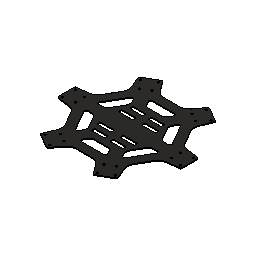
F550 Top Plate v11 (Autodesk Fusion 360 design; units mm, degrees)
Autodesk Fusion 360 part; units mm, degrees
sketch "Sketch1" plane through (0, 0, 0) normal (0, 0, 1) x (1, 0, 0)
  circle A0 centre (0, 0) radius 275 construction
  line L0 (-110, -15.85) -> (-110, 15.85)
  circle A1 centre (-105, 11.7505) radius 1.75
  circle A2 centre (-105, -11.7505) radius 1.75
  line L1 (-105, 11.7505) -> (-105, -11.7505) construction
  line L2 (0, 0) -> (-67.55, 39)
  line L3 (0, 0) -> (-67.55, -39)
  line L4 (0, 0) -> (-105, 0) construction
  line L5 (-110, -15.85) -> (-87.3993, -18.5941)
  line L6 (-67.55, -39) -> (-74.3532, -27.2165)
  arc A3 (-74.3532, -27.2165) -> (-87.3993, -18.5941) centre (-89.5086, -35.9665) ccw
  line L7 (-110, 15.85) -> (-87.3993, 18.5941)
  arc A4 (-87.3993, 18.5941) -> (-74.3532, 27.2165) centre (-89.5086, 35.9665) ccw
  line L8 (-67.55, 39) -> (-74.3532, 27.2165)
  circle A5 centre (-85.5, 8) radius 1.75
  circle A6 centre (-85.5, -8) radius 1.75
  line L9 (-85.5, -8) -> (-85.5, 8)
  line L10 (-54.5596, 31.5) -> (-64.5596, 14.1795)
  line L11 (-41.5692, 24) -> (-46.9504, 14.6795)
  line L12 (-61.9615, 9.6795) -> (-55.6107, 9.6795)
  arc A7 (-55.6107, 9.6795) -> (-46.9504, 14.6795) centre (-55.6107, 19.6795) ccw
  arc A8 (-64.5596, 14.1795) -> (-61.9615, 9.6795) centre (-61.9615, 12.6795) ccw
  line L13 (-54.5596, -31.5) -> (-64.5596, -14.1795)
  arc A9 (-61.9615, -9.6795) -> (-64.5596, -14.1795) centre (-61.9615, -12.6795) ccw
  line L14 (-61.9615, -9.6795) -> (-55.6107, -9.6795)
  arc A10 (-46.9504, -14.6795) -> (-55.6107, -9.6795) centre (-55.6107, -19.6795) ccw
  line L15 (-41.5692, -24) -> (-46.9504, -14.6795)
  point P0 (-110, 0)
  point P1 (-105, 0)
  point P2 (-275, 0)
  point P3 (-85.5, 0)
  point P4 (-107, -10)
  point P5 (-107, 10)
  point P6 (-107, 0)
  dimension "d1" = 550
  dimension "d2" = 23.501
  dimension "d3" = 5
  dimension "d5" = 170
  dimension "d6" = 3.5
  dimension "d7" = 31.7
  dimension "d8" = 30
  dimension "d9" = 30
  dimension "d10" = 78
  dimension "d11" = 16
  dimension "d12" = 19.5
  dimension "d13" = 20
  dimension "d23" = 3
  dimension "d24" = 10
  dimension "d25" = 15
  dimension "d26" = 60
  dimension "d28" = 15
  dimension "d29" = 20
  dimension "d30" = 105
  dimension "d31" = 23.359
  dimension "d44" = 17.5
  constraint coincident A0.centre L2.start
  constraint vertical L0
  constraint midpoint L0 P0
  constraint horizontal A0.centre P0
  constraint vertical A1.centre A2.centre
  constraint coincident A1.centre L1.start
  constraint coincident A2.centre L1.end
  constraint midpoint L1 P1
  constraint coincident A0 P2
  constraint horizontal A0.centre P2
  constraint equal A1 A2
  constraint coincident P1 L4.end
  constraint horizontal A0.centre P1
  constraint equal L2 L3
  constraint perpendicular L3 L6
  constraint tangent L6 A3
  constraint tangent L5 A3
  constraint symmetric L0.start L4 L0.end
  constraint symmetric L3.end L4 L2.end
  constraint symmetric L4 L5.end L7.end
  constraint symmetric L4 L6.end A4.end
  constraint symmetric L4 A3 A4
  constraint equal A5 A6
  constraint equal A1 A5
  constraint coincident A6.centre L9.start
  constraint coincident A5.centre L9.end
  constraint vertical L9
  constraint midpoint L9 P3
  constraint coincident L4 P3
  constraint coincident L2 L10.start
  constraint perpendicular L2 L10
  constraint coincident L2 L11.start
  constraint perpendicular L2 L11
  constraint tangent L11 A7
  constraint tangent L12 A8
  constraint tangent L10 A8
  constraint tangent L12 A7
  constraint symmetric L4 L10.start L13.start
  constraint symmetric L4 L10.end L13.end
  constraint symmetric L4 L11.start L15.start
  constraint symmetric L4 L11.end A10.start
  constraint symmetric L4 L12.start A9.start
  constraint symmetric L4 L12.end L14.end
  constraint symmetric L4 A7 A10
  constraint symmetric L4 A8 A9
  constraint coincident L4 P6
  measures "d1" diameter of A0
  measures "d2" distance of A1.centre A2.centre
  measures "d3" distance of L0 L1
  measures "d5" distance of L1 P2
  measures "d6" diameter of A1
  measures "d7" distance of L0.start L0.end
  measures "d8" angle of L3 L4
  measures "d9" angle of L2 L4
  measures "d10" distance of A0.centre L2.end
  measures "d11" distance of A6.centre A5.centre
  measures "d12" distance of L1 L9
  measures "d13" distance of P4 P5
  measures "d23" radius of A8
  measures "d24" radius of A7
  measures "d25" distance of L10 L11
  measures "d26" angle of L10 L12
  measures "d28" distance of L8 L10
  measures "d29" distance of L2 L10.end
  measures "d30" distance of L1 A0.centre
  measures "d44" radius of A4
extrude "Extrude1" add sketch "Sketch1" along normal blind 1.5 contours L0 L2 L3 L5 L6 A3 L7 A4 L8 L10 L11 L12 A7 A8 L13 A9 L14 A10 L15 makes body 1
fillet "Fillet1" radius 2 2 edges at (-110, 15.85, 0.75) (-110, -15.85, 0.75) on bodies 1
pattern_circular "C-Pattern1" count 6 over 360 about axis through (0, 0, 1.75) along (0, 0, 1) of bodies 1 makes body 2 at (-15.6501, -27.1068, 0) makes body 3 at (15.6501, -27.1068, 0) makes body 4 at (31.3003, 0, 1.5) makes body 5 at (15.6501, 27.1068, 0) makes body 6 at (-15.6501, 27.1068, 0)
combine "Combine1" operation add target body 1 tool bodies 2 3 4 5 6
sketch "Sketch2" plane through (0, 0, 1.5) normal (0, 0, 1) x (-1, 0, 0)
  line L0 (36.188, -33.3205) -> (46.9504, -14.6795)
  arc A0 (55.6107, -9.6795) -> (46.9504, -14.6795) centre (55.6107, -19.6795) ccw
  line L1 (55.6107, -9.6795) -> (61.9615, -9.6795)
  arc A1 (64.5596, -14.1795) -> (61.9615, -9.6795) centre (61.9615, -12.6795) ccw
  line L2 (64.5596, -14.1795) -> (44.5596, -48.8205)
  arc A2 (39.3634, -48.8205) -> (44.5596, -48.8205) centre (41.9615, -47.3205) ccw
  line L3 (39.3634, -48.8205) -> (36.188, -43.3205)
  arc A3 (36.188, -33.3205) -> (36.188, -43.3205) centre (44.8483, -38.3205) ccw
  line L4 (-10.7624, -48) -> (10.7624, -48)
  arc A4 (19.4226, -53) -> (10.7624, -48) centre (10.7624, -58) ccw
  line L5 (19.4226, -53) -> (22.5981, -58.5)
  arc A5 (20, -63) -> (22.5981, -58.5) centre (20, -60) ccw
  line L6 (20, -63) -> (-20, -63)
  circle A6 centre (49.6782, -70.0452) radius 1.75
  circle A7 centre (35.8218, -78.0452) radius 1.75
  circle A8 centre (62.6762, -85.0574) radius 1.75
  circle A9 centre (42.3238, -96.8079) radius 1.75
  line L7 (-13.6064, -78) -> (13.6064, -78)
  arc A10 (27.5967, -84.9871) -> (13.6064, -78) centre (13.6064, -95.5) ccw
  line L8 (27.5967, -84.9871) -> (40.2091, -101.7713)
  arc A11 (40.2091, -101.7713) -> (42.808, -102.3019) centre (41.808, -100.5698) ccw
  line L9 (42.808, -102.3019) -> (67.192, -88.2237)
  arc A12 (67.192, -88.2237) -> (68.032, -85.7077) centre (66.192, -86.4917) ccw
  line L10 (68.032, -85.7077) -> (59.8026, -66.393)
  arc A13 (60.7468, -50.7835) -> (59.8026, -66.393) centre (75.9022, -59.5335) ccw
  line L11 (60.7468, -50.7835) -> (74.3532, -27.2165)
  arc A14 (87.3993, -18.5941) -> (74.3532, -27.2165) centre (89.5086, -35.9665) ccw
  line L12 (87.3993, -18.5941) -> (108.2411, -16.0636)
  arc A15 (108.2411, -16.0636) -> (110, -14.0781) centre (108, -14.0781) ccw
  line L13 (110, -14.0781) -> (110, 14.0781)
  arc A16 (110, 14.0781) -> (108.2411, 16.0636) centre (108, 14.0781) ccw
  line L14 (108.2411, 16.0636) -> (87.3993, 18.5941)
  arc A17 (74.3532, 27.2165) -> (87.3993, 18.5941) centre (89.5086, 35.9665) ccw
  line L15 (74.3532, 27.2165) -> (60.7468, 50.7835)
  arc A18 (59.8026, 66.393) -> (60.7468, 50.7835) centre (75.9022, 59.5335) ccw
  line L16 (59.8026, 66.393) -> (68.032, 85.7077)
  arc A19 (68.032, 85.7077) -> (67.192, 88.2237) centre (66.192, 86.4917) ccw
  line L17 (67.192, 88.2237) -> (42.808, 102.3019)
  arc A20 (42.808, 102.3019) -> (40.2091, 101.7713) centre (41.808, 100.5698) ccw
  line L18 (40.2091, 101.7713) -> (27.5967, 84.9871)
  arc A21 (13.6064, 78) -> (27.5967, 84.9871) centre (13.6064, 95.5) ccw
  line L19 (13.6064, 78) -> (-13.6064, 78)
  arc A22 (-27.5967, 84.9871) -> (-13.6064, 78) centre (-13.6064, 95.5) ccw
  line L20 (-27.5967, 84.9871) -> (-40.2091, 101.7713)
  arc A23 (-40.2091, 101.7713) -> (-42.808, 102.3019) centre (-41.808, 100.5698) ccw
  line L21 (-42.808, 102.3019) -> (-67.192, 88.2237)
  arc A24 (-67.192, 88.2237) -> (-68.032, 85.7077) centre (-66.192, 86.4917) ccw
  line L22 (-68.032, 85.7077) -> (-59.8026, 66.393)
  arc A25 (-60.7468, 50.7835) -> (-59.8026, 66.393) centre (-75.9022, 59.5335) ccw
  line L23 (-60.7468, 50.7835) -> (-74.3532, 27.2165)
  arc A26 (-87.3993, 18.5941) -> (-74.3532, 27.2165) centre (-89.5086, 35.9665) ccw
  line L24 (-87.3993, 18.5941) -> (-108.2411, 16.0636)
  arc A27 (-108.2411, 16.0636) -> (-110, 14.0781) centre (-108, 14.0781) ccw
  line L25 (-110, 14.0781) -> (-110, -14.0781)
  arc A28 (-110, -14.0781) -> (-108.2411, -16.0636) centre (-108, -14.0781) ccw
  line L26 (-108.2411, -16.0636) -> (-87.3993, -18.5941)
  arc A29 (-74.3532, -27.2165) -> (-87.3993, -18.5941) centre (-89.5086, -35.9665) ccw
  line L27 (-74.3532, -27.2165) -> (-60.7468, -50.7835)
  arc A30 (-59.8026, -66.393) -> (-60.7468, -50.7835) centre (-75.9022, -59.5335) ccw
  line L28 (-59.8026, -66.393) -> (-68.032, -85.7077)
  arc A31 (-68.032, -85.7077) -> (-67.192, -88.2237) centre (-66.192, -86.4917) ccw
  line L29 (-67.192, -88.2237) -> (-42.808, -102.3019)
  arc A32 (-42.808, -102.3019) -> (-40.2091, -101.7713) centre (-41.808, -100.5698) ccw
  line L30 (-40.2091, -101.7713) -> (-27.5967, -84.9871)
  arc A33 (-13.6064, -78) -> (-27.5967, -84.9871) centre (-13.6064, -95.5) ccw
  circle A34 centre (-35.8218, -78.0452) radius 1.75
  circle A35 centre (-49.6782, -70.0452) radius 1.75
  circle A36 centre (-42.3238, -96.8079) radius 1.75
  circle A37 centre (-62.6762, -85.0574) radius 1.75
  circle A38 centre (-85.5, -8) radius 1.75
  circle A39 centre (-85.5, 8) radius 1.75
  circle A40 centre (-105, -11.7505) radius 1.75
  circle A41 centre (-105, 11.7505) radius 1.75
  circle A42 centre (-49.6782, 70.0452) radius 1.75
  circle A43 centre (-35.8218, 78.0452) radius 1.75
  circle A44 centre (-62.6762, 85.0574) radius 1.75
  circle A45 centre (-42.3238, 96.8079) radius 1.75
  line L31 (10.7624, 48) -> (-10.7624, 48)
  arc A46 (-19.4226, 53) -> (-10.7624, 48) centre (-10.7624, 58) ccw
  line L32 (-19.4226, 53) -> (-22.5981, 58.5)
  arc A47 (-20, 63) -> (-22.5981, 58.5) centre (-20, 60) ccw
  line L33 (-20, 63) -> (20, 63)
  arc A48 (22.5981, 58.5) -> (20, 63) centre (20, 60) ccw
  line L34 (22.5981, 58.5) -> (19.4226, 53)
  arc A49 (10.7624, 48) -> (19.4226, 53) centre (10.7624, 58) ccw
  circle A50 centre (35.8218, 78.0452) radius 1.75
  circle A51 centre (49.6782, 70.0452) radius 1.75
  circle A52 centre (42.3238, 96.8079) radius 1.75
  circle A53 centre (62.6762, 85.0574) radius 1.75
  line L35 (46.9504, 14.6795) -> (36.188, 33.3205)
  arc A54 (36.188, 43.3205) -> (36.188, 33.3205) centre (44.8483, 38.3205) ccw
  line L36 (36.188, 43.3205) -> (39.3634, 48.8205)
  arc A55 (44.5596, 48.8205) -> (39.3634, 48.8205) centre (41.9615, 47.3205) ccw
  line L37 (44.5596, 48.8205) -> (64.5596, 14.1795)
  arc A56 (61.9615, 9.6795) -> (64.5596, 14.1795) centre (61.9615, 12.6795) ccw
  line L38 (61.9615, 9.6795) -> (55.6107, 9.6795)
  arc A57 (46.9504, 14.6795) -> (55.6107, 9.6795) centre (55.6107, 19.6795) ccw
  circle A58 centre (105, -11.7505) radius 1.75
  circle A59 centre (105, 11.7505) radius 1.75
  circle A60 centre (85.5, -8) radius 1.75
  circle A61 centre (85.5, 8) radius 1.75
  line L39 (32, -16) -> (9, -16)
  line L40 (8, -17) -> (8, -21)
  line L41 (9, -22) -> (32, -22)
  line L42 (33, -21) -> (33, -17)
  line L43 (27, -31) -> (6, -31)
  line L44 (5, -32) -> (5, -36)
  line L45 (6, -37) -> (27, -37)
  line L46 (28, -36) -> (28, -32)
  line L47 (0, 0) -> (0, -78) construction
  line L48 (0, 0) -> (110, 0) construction
  arc A62 (27, -37) -> (28, -36) centre (27, -36) ccw
  arc A63 (5, -36) -> (6, -37) centre (6, -36) ccw
  arc A64 (6, -31) -> (5, -32) centre (6, -32) ccw
  arc A65 (28, -32) -> (27, -31) centre (27, -32) ccw
  arc A66 (32, -22) -> (33, -21) centre (32, -21) ccw
  arc A67 (8, -21) -> (9, -22) centre (9, -21) ccw
  arc A68 (9, -16) -> (8, -17) centre (9, -17) ccw
  arc A69 (33, -17) -> (32, -16) centre (32, -17) ccw
  arc A70 (-27, -31) -> (-28, -32) centre (-27, -32) ccw
  arc A71 (-28, -36) -> (-27, -37) centre (-27, -36) ccw
  line L49 (-6, -37) -> (-27, -37)
  line L50 (-9, -22) -> (-32, -22)
  arc A72 (-33, -21) -> (-32, -22) centre (-32, -21) ccw
  arc A73 (-5, -32) -> (-6, -31) centre (-6, -32) ccw
  arc A74 (-6, -37) -> (-5, -36) centre (-6, -36) ccw
  line L51 (-28, -36) -> (-28, -32)
  arc A75 (-8, -17) -> (-9, -16) centre (-9, -17) ccw
  arc A76 (-9, -22) -> (-8, -21) centre (-9, -21) ccw
  line L52 (-32, -16) -> (-9, -16)
  arc A77 (-32, -16) -> (-33, -17) centre (-32, -17) ccw
  line L53 (-8, -17) -> (-8, -21)
  line L54 (-5, -32) -> (-5, -36)
  line L55 (-27, -31) -> (-6, -31)
  line L56 (-33, -21) -> (-33, -17)
  line L57 (27, 31) -> (6, 31)
  line L58 (-8, 17) -> (-8, 21)
  arc A78 (8, 17) -> (9, 16) centre (9, 17) ccw
  arc A79 (9, 22) -> (8, 21) centre (9, 21) ccw
  line L59 (-33, 21) -> (-33, 17)
  line L60 (33, 21) -> (33, 17)
  line L61 (-27, 31) -> (-6, 31)
  line L62 (-5, 32) -> (-5, 36)
  arc A80 (-9, 16) -> (-8, 17) centre (-9, 17) ccw
  line L63 (-28, 36) -> (-28, 32)
  arc A81 (27, 31) -> (28, 32) centre (27, 32) ccw
  arc A82 (28, 36) -> (27, 37) centre (27, 36) ccw
  line L64 (-32, 16) -> (-9, 16)
  line L65 (32, 16) -> (9, 16)
  line L66 (-6, 37) -> (-27, 37)
  arc A83 (-32, 22) -> (-33, 21) centre (-32, 21) ccw
  arc A84 (5, 32) -> (6, 31) centre (6, 32) ccw
  arc A85 (-8, 21) -> (-9, 22) centre (-9, 21) ccw
  arc A86 (-5, 36) -> (-6, 37) centre (-6, 36) ccw
  line L67 (-9, 22) -> (-32, 22)
  arc A87 (-33, 17) -> (-32, 16) centre (-32, 17) ccw
  line L68 (5, 32) -> (5, 36)
  arc A88 (33, 21) -> (32, 22) centre (32, 21) ccw
  line L69 (9, 22) -> (32, 22)
  arc A89 (-6, 31) -> (-5, 32) centre (-6, 32) ccw
  arc A90 (6, 37) -> (5, 36) centre (6, 36) ccw
  line L70 (8, 17) -> (8, 21)
  line L71 (28, 36) -> (28, 32)
  line L72 (6, 37) -> (27, 37)
  arc A91 (32, 16) -> (33, 17) centre (32, 17) ccw
  arc A92 (-27, 37) -> (-28, 36) centre (-27, 36) ccw
  arc A93 (-28, 32) -> (-27, 31) centre (-27, 32) ccw
  point P0 (33, -16)
  point P1 (8, -16)
  point P2 (28, -31)
  point P3 (5, -37)
  point P4 (28, -37)
  point P5 (-8, -16)
  point P6 (-33, -16)
  point P7 (-28, -37)
  point P8 (-28, -31)
  point P9 (-5, -37)
  point P10 (-28, 37)
  point P11 (-5, 37)
  point P12 (-33, 16)
  point P13 (5, 37)
  point P14 (-28, 31)
  point P15 (28, 37)
  point P16 (-8, 16)
  point P17 (8, 16)
  point P18 (28, 31)
  point P19 (33, 16)
  dimension "d33" = 5
  dimension "d34" = 8
  dimension "d35" = 16
  dimension "d36" = 9
  dimension "d38" = 23
  dimension "d39" = 25
  dimension "d40" = 1
  dimension "d41" = 1
  dimension "d42" = 6
  constraint horizontal L39
  constraint vertical L40
  constraint horizontal L41
  constraint vertical L42
  constraint horizontal L43
  constraint vertical L44
  constraint horizontal L45
  constraint vertical L46
  constraint equal L42 L46
  constraint coincident L47.start L48.start
  constraint midpoint L7 L47.end
  constraint midpoint L13 L48.end
  constraint coincident P4 L46
  constraint coincident P4 L45
  constraint tangent L46 A62
  constraint tangent L45 A62
  constraint coincident P3 L45
  constraint coincident P3 L44
  constraint tangent L45 A63
  constraint tangent L44 A63
  constraint equal A62 A63
  constraint tangent L43 A64
  constraint tangent L44 A64
  constraint equal A62 A64
  constraint coincident P2 L43
  constraint coincident P2 L46
  constraint tangent L43 A65
  constraint tangent L46 A65
  constraint equal A62 A65
  constraint tangent L42 A66
  constraint tangent L41 A66
  constraint tangent L41 A67
  constraint tangent L40 A67
  constraint equal A66 A67
  constraint coincident P1 L39
  constraint coincident P1 L40
  constraint tangent L39 A68
  constraint tangent L40 A68
  constraint equal A66 A68
  constraint coincident P0 L39
  constraint coincident P0 L42
  constraint tangent L39 A69
  constraint tangent L42 A69
  constraint equal A66 A69
  constraint symmetric P0 L47 P6
  constraint symmetric P1 L47 P5
  constraint symmetric P2 L47 P8
  constraint symmetric P3 L47 P9
  constraint symmetric P4 L47 P7
  constraint symmetric L47 L46.start A71.start
  constraint symmetric L47 L45.end A71.end
  constraint symmetric L47 A62 A71
  constraint symmetric L47 L45.start L49.start
  constraint symmetric L47 L44.end A74.end
  constraint symmetric L47 A63 A74
  constraint symmetric L47 L43.end A73.end
  constraint symmetric L47 L44.start A73.start
  constraint symmetric L47 A64 A73
  constraint symmetric L47 L43.start A70.start
  constraint symmetric L47 L46.end A70.end
  constraint symmetric L47 A65 A70
  constraint symmetric L47 L42.start A72.start
  constraint symmetric L47 L41.end L50.end
  constraint symmetric L47 A66 A72
  constraint symmetric L47 L41.start L50.start
  constraint symmetric L47 L40.end A76.end
  constraint symmetric L47 A67 A76
  constraint symmetric L47 L39.end A75.end
  constraint symmetric L47 L40.start A75.start
  constraint symmetric L47 A68 A75
  constraint symmetric L47 L39.start L52.start
  constraint symmetric L47 L42.end A77.end
  constraint symmetric L47 A69 A77
  constraint symmetric P0 L48 P19
  constraint symmetric P1 L48 P17
  constraint symmetric P2 L48 P18
  constraint symmetric P3 L48 P13
  constraint symmetric P4 L48 P15
  constraint symmetric L48 L46.start A82.start
  constraint symmetric L48 L45.end A82.end
  constraint symmetric L48 A62 A82
  constraint symmetric L48 L45.start A90.start
  constraint symmetric L48 L44.end L68.end
  constraint symmetric L48 A63 A90
  constraint symmetric L48 L43.end L57.end
  constraint symmetric L48 L44.start A84.start
  constraint symmetric L48 A64 A84
  constraint symmetric L48 L43.start L57.start
  constraint symmetric L48 L46.end A81.end
  constraint symmetric L48 A65 A81
  constraint symmetric L48 L42.start L60.start
  constraint symmetric L48 L41.end A88.end
  constraint symmetric L48 A66 A88
  constraint symmetric L48 L41.start A79.start
  constraint symmetric L48 L40.end A79.end
  constraint symmetric L48 A67 A79
  constraint symmetric L48 L39.end A78.end
  constraint symmetric L48 L40.start A78.start
  constraint symmetric L48 A68 A78
  constraint symmetric L48 L39.start L65.start
  constraint symmetric L48 L42.end L60.end
  constraint symmetric L48 A69 A91
  constraint symmetric L48 L49.start L66.start
  constraint symmetric L48 P5 P16
  constraint symmetric L48 A71.end L66.end
  constraint symmetric L48 A74.end L62.end
  constraint symmetric L48 P6 P12
  constraint symmetric L48 L50.end A83.start
  constraint symmetric L48 P7 P10
  constraint symmetric L48 L50.start A85.end
  constraint symmetric L48 A76.end L58.end
  constraint symmetric L48 A72.start L59.start
  constraint symmetric L48 A77.end L59.end
  constraint symmetric L48 A71.start L63.start
  constraint symmetric L48 A75.start L58.start
  constraint symmetric L48 L52.start L64.start
  constraint symmetric L48 A75.end A80.start
  constraint symmetric L48 A70.start L61.start
  constraint symmetric L48 A73.start L62.start
  constraint symmetric L48 P8 P14
  constraint symmetric L48 P9 P11
  constraint symmetric L48 A73.end L61.end
  constraint symmetric L48 A70.end L63.end
  constraint symmetric L48 A70 A93
  constraint symmetric L48 A71 A92
  constraint symmetric L48 A72 A83
  constraint symmetric L48 A73 A89
  constraint symmetric L48 A74 A86
  constraint symmetric L48 A75 A80
  constraint symmetric L48 A76 A85
  constraint symmetric L48 A77 A87
  measures "d33" distance of L47.start L44
  measures "d34" distance of L47.start L40
  measures "d35" distance of L47.start L39
  measures "d38" distance of P3 P4
  measures "d39" distance of P0 P1
  measures "d40" radius of A62
  measures "d42" distance of L43 L45
extrude "Extrude2" cut sketch "Sketch2" against normal through all contours L39 L40 L41 L42 A66 A67 A68 A69 | L43 L44 L45 L46 A62 A63 A64 A65 | A70 A71 L49 A73 A74 L51 L54 L55 | L50 A72 A75 A76 L52 A77 L53 L56 | L57 A81 A82 A84 L68 A90 L71 L72 | L58 L59 A80 L64 A83 A85 L67 A87 | A78 A79 L60 L65 A88 L69 L70 A91 | L61 L62 L63 L66 A86 A89 A92 A93 bodies 1
equation "d9 = d8"
equation "d10 = ( 156 / 2 ) * 1 mm"
equation "d35 = ( 32 / 2 ) * 1 mm"
